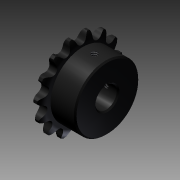
# Autodesk Inventor part: 36684074
Saved by Autodesk Inventor 2011 (Build 150239000, 239)
## iProperties
Created: 2008-12-11
Part Number: 36684074
Material: Steel
Document SubType Name: Modeling
Designer: Autodesk Inc.
Density: 1 g/cm^3
Catalog Web Link: http://www1.mscdirect.com/CGI/NNSRIT?PMAKA=36684074
Vendor: MSC Direct
Description: Roller Chain Sprockets Teeth: 15 Size: 35 Chain Pitch: 3/8
CustomPartVersion: 1
Category: Drive Train
Company: Autodesk Inc.
Author: Autodesk Inc.
Autodesk Inventor part; units mm, degrees
ref_plane "YZ Plane" through (0, 0, 0) normal (1, 0, 0) x (0, 1, 0)
sketch "Theoretical Tooth Profile" plane through (0, 0, 0) normal (0, 0, 1) x (1, 0, 0)
  circle A0 centre (0, 0) radius 22.9064 construction
  line L0 (0, 0) -> (0, 22.9064) construction
  line L1 (0, 0) -> (9.3169, 20.926) construction
  circle A1 centre (0, 0) radius 25.2633
  arc A2 (-2.0134, 21.2759) -> (2.0134, 21.2759) centre (0, 22.9064) ccw
  line L2 (0, 22.9064) -> (9.3169, 20.926) construction
  line L3 (0, 22.9064) -> (3.1583, 25.4639) construction
  line L4 (3.1583, 25.4639) -> (-2.886, 22.6796) construction
  arc A3 (4.4991, 24.8595) -> (3.1228, 23.1937) centre (6.9566, 21.4277) ccw
  arc A4 (-3.1228, 23.1937) -> (-4.4991, 24.8595) centre (-6.9566, 21.4277) ccw
  line L5 (-6.9566, 21.4277) -> (-3.1228, 23.1937) construction
  arc A5 (-2.886, 22.6796) -> (-2.0134, 21.2759) centre (3.1583, 25.4639) ccw
  line L6 (-2.886, 22.6796) -> (-3.1228, 23.1937)
  arc A6 (2.0134, 21.2759) -> (2.886, 22.6796) centre (-3.1583, 25.4639) ccw
  line L7 (3.1228, 23.1937) -> (2.886, 22.6796)
  line L8 (0, 0) -> (5.2525, 24.7112) construction
  point P0 (4.6584, 21.9162)
  dimension "d0" = 45.8127
  dimension "d2" = 24
  dimension "d3" = 2.5908
  dimension "d10" = 129
  dimension "d11" = 14.267
  dimension "d12" = 4.064
  dimension "d13" = 6.6548
  dimension "d14" = 7.112
  dimension "d23" = 2.8575
  constraints: 18 end point, 15 point on circle, 7 centre point, 3 coincident, 3 point on line, 3 symmetric about line, 3 tangent, 1 equal radius, 1 midpoint, 1 parallel, 1 vertical, 1 other
  measures "d0" diameter of A0
  measures "d2" angle of L1 L0
  measures "d3" radius of A2
  measures "d10" angle of L3 L0
  measures "d11" angle of L4 L3
  measures "d12" distance of L2.start L3.end
  measures "d13" distance of L3.end L4.end
  measures "d14" distance of A3.centre L0.end
  measures "d23" distance from line of L8.end L2
sketch "Tooth Profile" plane through (0, 0, 0) normal (0, 0, 1) x (1, 0, 0)
  circle A0 centre (0, 0) radius 25.2633 projected
  line L0 (0, 0) -> (0, 22.9064) construction
  line L1 (0, 22.9064) -> (2.3848, 21.8941) construction
  arc A1 (-2.3848, 21.8941) -> (2.3848, 21.8941) centre (0, 22.9064) ccw
  line L2 (-2.3848, 21.8941) -> (0, 22.9064) construction
  arc A2 (-2.3848, 21.8941) -> (-4.3245, 24.8904) centre (-11.9242, 17.8448) ccw
  arc A3 (4.3245, 24.8904) -> (2.3848, 21.8941) centre (11.9242, 17.8448) ccw
  dimension "d44" = 134
  dimension "d45" = 2.5908
  dimension "d46" = 10.3632
  constraints: 8 point on circle, 7 end point, 3 centre point, 2 tangent, 1 coincident, 1 equal radius, 1 symmetric about line, 1 vertical
  measures "d44" angle of L1 L2
  measures "d45" radius of A1
  measures "d46" radius of A3
sketch "Section Profile" plane through (0, 0, 0) normal (1, 0, 0) x (0, 1, 0)
  line L0 (25.2633, 0) -> (-25.2633, 0) projected
  line L1 (16.8813, 2.2967) -> (-16.8813, 2.2967)
  line L2 (-16.8813, 2.2967) -> (-16.8813, -2.2967)
  line L3 (-16.8813, -2.2967) -> (16.8813, -2.2967)
  line L4 (16.8813, -2.2967) -> (16.8813, 2.2967)
  line L5 (16.8813, 2.2967) -> (25.2633, 2.2967) construction
  line L6 (25.2633, 2.2967) -> (25.2633, -2.2967) construction
  line L7 (25.2633, -2.2967) -> (16.8813, -2.2967) construction
  line L8 (16.8813, -2.2967) -> (16.8813, 2.2967)
  arc A0 (25.2633, 1.106) -> (20.4996, 2.2967) centre (20.4996, -7.8284) ccw
  arc A1 (20.4996, -2.2967) -> (25.2633, -1.106) centre (20.4996, 7.8284) ccw
  line L9 (20.4996, 2.2967) -> (0, 2.2967)
  line L10 (0, 2.2967) -> (0, -2.2967)
  line L11 (0, -2.2967) -> (20.4996, -2.2967)
  line L12 (0, 2.2967) -> (0, -2.2967)
  line L13 (25.2633, 1.106) -> (25.2633, -1.106)
  point P0 (0, 0)
  point P1 (0, 0)
  dimension "d30" = 4.5933
  dimension "d31" = 33.7626
  dimension "d32" = 4.5933
  dimension "d33" = 1.1906
  dimension "d34" = 10.1251
  dimension "d43" = 2.2967
  constraints: 26 end point, 7 midpoint, 5 perpendicular, 4 parallel, 4 point on circle, 3 point on line, 3 symmetric about line, 2 centre point, 2 horizontal, 2 tangent, 1 collinear, 1 other
  measures "d30" distance between parallel lines of L7 L5
  measures "d31" distance between parallel lines of L2 L4
  measures "d32" distance between parallel lines of L3 L1
  measures "d33" distance from line of L13.start L5
  measures "d34" radius of A0
  measures "d43" distance between parallel lines of L3 L0
revolve "Shroud" add sketch "Section Profile" angle 360 about axis through (0, 0, 2.2967) along (0, 0, -1) contours L10 L3 L2 L0 | L0 L2 L1 L10
revolve "Strand" add sketch "Section Profile" angle 360 about axis through (0, 0, 2.2967) along (0, 0, -1) contours L13 A1 L11 L4 L0 | L0 L4 L9 A0 L13 | L4 L3 L10 L0 | L0 L10 L1 L4
pattern_of_one "Strand Pattern"
extrude "Theoretical Tooth" cut sketch "Theoretical Tooth Profile" along normal through all both and the other way through all contours A3 L7 A6 A2 A5 L6 A4 A1 picked at (-0.5023, 22.59)
extrude "Tooth" [suppressed]
pattern_circular "Tooth Pattern" count 15 over 360 about axis through (0, 0, -10) along (0, 0, 1) of "Theoretical Tooth"
ref_plane "Timing Plane" through (0, 22.9064, 0) normal (1, 0, 0) x (0, 1, 0)
sketch "Sketch4" plane through (0, 22.9064, 2.2967) normal (0, 0, 1) x (1, 0, 0)
  circle A0 centre (0.6902, -22.9064) radius 19.05
  dimension "d51" = 38.1
  constraints: 1 centre point
  measures "d51" diameter of A0
extrude "Extrusion4" add sketch "Sketch4" along normal blind 14.5313
sketch "Sketch5" plane through (0.6902, 0, 16.828) normal (0, 0, 1) x (1, 0, 0)
  circle A0 centre (0, 0) radius 19.05 projected
hole "Hole1" at (0.6902, 0, 16.828) direction (0, 0, -1) diameter 12.7 end up to surface
sketch "Sketch6" plane through (0.6902, 0, 16.828) normal (0, 0, 1) x (1, 0, 0)
  circle A0 centre (0, 0) radius 6.35 projected
  circle A1 centre (0, 0) radius 19.05 projected
  line L0 (-1.5875, 6.1484) -> (-1.5875, 7.874)
  line L1 (-1.5875, 7.874) -> (1.5875, 7.874)
  line L2 (1.5875, 7.874) -> (1.5875, 6.1484)
  line L3 (0, 0) -> (0, 6.35) construction
  point P0 (0, 7.874)
  dimension "d61" = 3.175
  dimension "d62" = 1.524
  constraints: 8 end point, 3 point on circle, 2 parallel, 1 midpoint, 1 perpendicular, 1 vertical, 1 vertical alignment
  measures "d61" distance of L0.end L1.end
  measures "d62" distance from line of L1 L3.end
extrude "Extrusion5" cut sketch "Sketch6" against normal up to next contours A0 L0 L1 L2
chamfer "Chamfer1" distance 0.7937 angle 45 1 edges at (-18.3598, 0, 16.828)
chamfer "Chamfer2" distance 0.7937 angle 45 2 edges at (0.6902, -6.35, 16.828) (0.6902, -6.35, -2.2967)
ref_plane "Work Plane3" through (0.6902, 19.05, 2.2967) normal (0, 1, 0) x (-1, 0, 0)
sketch "Sketch7" plane through (0.6902, 19.05, 2.2967) normal (0, 1, 0) x (-1, 0, 0)
  line L0 (-18.2563, 14.5313) -> (18.2563, 14.5313) projected
  point P0 (0, 6.9907)
  point P1 (0, 14.5313)
  dimension "d71" = 7.5406
  constraints: 1 midpoint, 1 vertical alignment
  measures "d71" distance from line of L0 point (0, 6.991)
hole "Hole2" at (0.6902, 19.05, 9.2874) direction (0, -1, 0) diameter 3.683 end up to surface thread size "10-24 UNC" class "2B" standard "ANSI Unified Screw Threads"
pattern_circular "Circular Pattern2" count 2 over 90 about axis through (0.6902, 0, 2.2967) along (0, 0, -1) of "Hole2"
equation "\"d3\" = 0.5 * da_Dr + da_SC"
equation "\"d12\" = 0.8 * da_Dr"
equation "\"d13\" = 1.3 * da_Dr + da_SC"
equation "\"d14\" = 1.4 * da_Dr"
equation "\"d23\" = da_Ha"
equation "\"d44\" = da_Alfa"
equation "\"d45\" = da_Ri"
equation "\"d46\" = da_Re"
equation "\"d30\" = da_Bf"
equation "\"d31\" = da_Ds"
equation "\"d32\" = da_Bs"
equation "\"d33\" = da_Ba"
equation "\"d34\" = da_Rx"
equation "\"d40\" = da_pt"
equation "\"form_type\" = 0"
equation "\"da_p\" = 9.525"
equation "\"da_Dr\" = 5.08"
equation "\"da_SC\" = 0.0508"
equation "\"da_Ha\" = 2.8575"
equation "\"da_pt\" = 10.1346"
equation "\"da_Bf\" = 4.59334"
equation "\"da_Ba\" = 1.19063"
equation "\"da_Rx\" = 10.12508"
equation "\"da_Ra\" = 0.381"
equation "\"da_Bs\" = 4.59334"
equation "\"da_Ds\" = 33.7626"
equation "\"da_Re\" = 10.3632"
equation "\"da_Ri\" = 2.5908"
equation "\"da_Alfa\" = 134deg"
body "Solid1"
